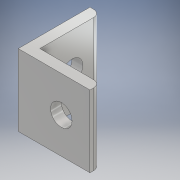
# Autodesk Inventor part: Cantoneira Gaveta
Saved by Autodesk Inventor 2018 (Build 220112000, 112)
## iProperties
Created: 2018-07-12
Part Number: Cantoneira Gaveta
Material: Liga de aço
Document SubType Name: Modeling
Designer: Regner
Density: 7.73 g/cm^3
Appearance: Alumínio - Polido
Author: Regner
Autodesk Inventor part; units mm, degrees
ref_plane "YZ Plane" through (0, 0, 0) normal (1, 0, 0) x (0, 1, 0)
ref_plane "XZ Plane" through (0, 0, 0) normal (0, 1, 0) x (-1, 0, 0)
ref_plane "XY Plane" through (0, 0, 0) normal (0, 0, 1) x (1, 0, 0)
sketch "Esboço1" plane through (0, 0, 0) normal (0, 0, 1) x (1, 0, 0)
  line L0 (5, -5) -> (-5, -5)
  line L1 (-5, -5) -> (-5, 5)
  line L2 (-5, 5) -> (-3.5, 5)
  line L3 (5, -3.5) -> (5, -5)
  line L4 (5, -5) -> (-5, 5) construction
  line L5 (-5, -5) -> (5, 5) construction
  line L6 (-3.5, 5) -> (-3.5, -3.5)
  line L7 (5, -3.5) -> (-3.5, -3.5)
  point P0 (0, 0)
  dimension "d0" = 10
  dimension "d1" = 10
  dimension "d2" = 1.5
  dimension "d4" = 5
  dimension "d5" = 5
  constraints: 16 end point, 2 midpoint, 2 parallel, 2 perpendicular, 1 horizontal, 1 point on line, 1 vertical
  measures "d0" distance of L1.end L5.end
  measures "d1" distance of L0.end L1.end
  measures "d2" distance between parallel lines of L1 L6
  measures "d4" distance from line of point (0, 0) L1
  measures "d5" distance from line of point (0, 0) L0
extrude "Extrusão1" add sketch "Esboço1" along normal mid plane 10
fillet "Arredondamento1" radius 1 2 edges at (-3.5, 5, 0) (5, -3.5, 0)
hole "Furo1" at (1, -3.5, 0) direction (0, -1, 0) diameter 3 end through all
hole "Furo2" at (-3.5, 1, 0) direction (-1, 0, 0) diameter 3 end through all
equation "\"d4\" = 0.5 * d0"
equation "\"d5\" = 0.5 * d1"
